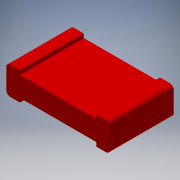
# Autodesk Inventor part: SPDT Toggle Switch Base
Saved by Autodesk Inventor 2016 (Build 200138000, 138)
## iProperties
Created: 2011-11-07
Part Number: SPDT Toggle Switch Base
Document SubType Name: Modeling
Designer: sdarley
Density: 1 g/cm^3
Material: Generic
Appearance: Red
Author: sdarley
Autodesk Inventor part; units mm, degrees
ref_plane "YZ Plane" through (0, 0, 0) normal (1, 0, 0) x (0, 1, 0)
ref_plane "XZ Plane" through (0, 0, 0) normal (0, 1, 0) x (-1, 0, 0)
ref_plane "XY Plane" through (0, 0, 0) normal (0, 0, 1) x (1, 0, 0)
sketch "Sketch1" plane through (0, 0, 0) normal (0, 0, 1) x (1, 0, 0)
  line L0 (-13, 8) -> (13, 8)
  line L1 (13, 8) -> (13, -8)
  line L2 (13, -8) -> (-13, -8)
  line L3 (-13, -8) -> (-13, 8)
  point P0 (0, 0)
  point P1 (-13, 0)
  point P2 (0, -8)
  dimension "d0" = 16
  dimension "d1" = 26
  constraints: 8 end point, 2 midpoint, 2 parallel, 1 horizontal, 1 horizontal alignment, 1 perpendicular, 1 vertical alignment
  measures "d0" distance between parallel lines of L0 L2
  measures "d1" distance between parallel lines of L1 L3
extrude "Extrusion1" add sketch "Sketch1" along normal blind 7
sketch "Sketch2" plane through (-13, 8, 0) normal (0, 1, 0) x (1, 0, 0)
  line L0 (0, -7) -> (26, -7) projected
  line L1 (0, 0) -> (26, 0) projected
  line L2 (22.55, -7) -> (3.45, -7)
  line L3 (3.45, -7) -> (3.45, -6)
  line L4 (3.45, -6) -> (22.55, -6)
  line L5 (22.55, -6) -> (22.55, -7)
  line L6 (22.55, 0) -> (3.45, 0)
  line L7 (3.45, 0) -> (3.45, -1)
  line L8 (3.45, -1) -> (22.55, -1)
  line L9 (22.55, -1) -> (22.55, 0)
  line L10 (1.725, -0.05) -> (11.275, -0.05) projected
  line L11 (1.725, -0.3) -> (1.725, -0.05) projected
  line L12 (0.5, -0.3) -> (1.725, -0.3) projected
  line L13 (0, -0.8) -> (0.5, -0.3) projected
  line L14 (0, -6.2) -> (0, -0.8) projected
  line L15 (0.5, -6.7) -> (0, -6.2) projected
  line L16 (1.725, -6.7) -> (0.5, -6.7) projected
  line L17 (1.725, -6.7) -> (1.725, -6.75) projected
  line L18 (11.275, -6.75) -> (1.725, -6.75) projected
  line L19 (11.275, -6.7) -> (11.275, -6.75) projected
  line L20 (12.5, -6.7) -> (11.275, -6.7) projected
  line L21 (13, -6.2) -> (12.5, -6.7) projected
  line L22 (13, -0.8) -> (13, -6.2) projected
  line L23 (12.5, -0.3) -> (13, -0.8) projected
  line L24 (11.275, -0.3) -> (12.5, -0.3) projected
  line L25 (11.275, -0.3) -> (11.275, -0.05) projected
  point P0 (13, 0)
  point P1 (13, -7)
  point P2 (13, -7)
  point P3 (13, -1)
  point P4 (13, 0)
  dimension "d4" = 1
  dimension "d5" = 1
  dimension "d6" = 19.1
  dimension "d7" = 19.1
  constraints: 16 end point, 4 midpoint, 4 parallel, 2 horizontal, 2 perpendicular, 2 point on line, 1 coincident, 1 vertical alignment
  measures "d4" distance of L2.end L3.end
  measures "d5" distance of L7.end L6.end
  measures "d6" distance between parallel lines of L3 L5
  measures "d7" distance between parallel lines of L7 L9
extrude "Extrusion2" cut sketch "Sketch2" against normal through all contours L3 L18 L19 L20 L21 L22 L4 L5 L0 | L3 L4 L22 L21 L20 L19 L18 | L22 L23 L24 L25 L10 L7 L1 L9 L8 | L8 L7 L10 L25 L24 L23 L22
fillet "Fillet1" radius 1 4 edges at (13, 0, 7) (13, 0, 0) (-13, 0, 0) (-13, 0, 7)
equation "\"d7\" = d6"
body "Solid1"
